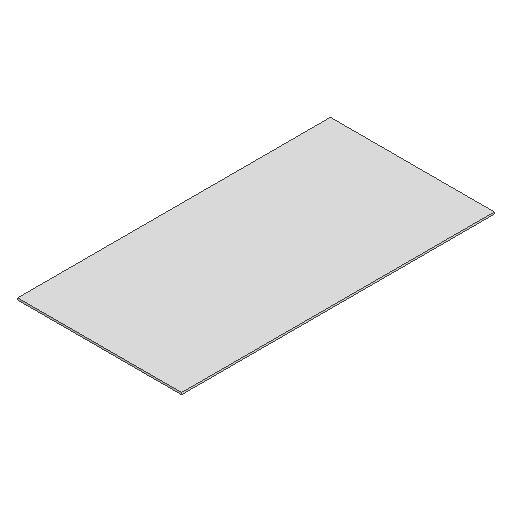
# Autodesk Inventor part: TableTop
Saved by Autodesk Inventor 2022 (Build 260148000, 148)
## iProperties
Created: 2021-03-15
Part Number: TableTop
Material: Generic
Document SubType Name: Modeling
Designer: jmacmillan
Density: 1 g/cm^3
Appearance: Default
Author: jmacmillan
Autodesk Inventor part; units mm, degrees
ref_plane "YZ Plane" through (0, 0, 0) normal (1, 0, 0) x (0, 1, 0)
ref_plane "XZ Plane" through (0, 0, 0) normal (0, 1, 0) x (-1, 0, 0)
ref_plane "XY Plane" through (0, 0, 0) normal (0, 0, 1) x (1, 0, 0)
sketch "Sketch1" plane through (0, 0, 0) normal (0, 1, 0) x (-1, 0, 0)
  line L0 (275.4, 525.4) -> (-275.4, 525.4)
  line L1 (-275.4, 525.4) -> (-275.4, -525.4)
  line L2 (-275.4, -525.4) -> (275.4, -525.4)
  line L3 (275.4, -525.4) -> (275.4, 525.4)
  line L4 (0, -735.56) -> (0, 735.56) projected
  line L5 (-385.56, 0) -> (385.56, 0) projected
  point P0 (0, 0)
  dimension "d0" = 1050.8
  dimension "d1" = 550.8
  constraints: 8 end point, 2 parallel, 1 horizontal, 1 perpendicular, 2 other
  measures "d0" distance of L2.end L0.start
  measures "d1" distance of L1.end L2.end
extrude "Extrusion1" add sketch "Sketch1" along normal blind 6.35
body "Solid1"
